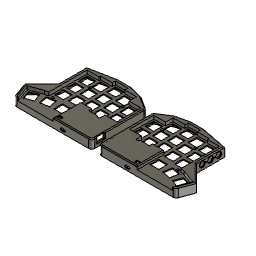
top_23333_3 (Autodesk Fusion 360 design; units mm, degrees)
Autodesk Fusion 360 part; units mm, degrees
sketch "case_plate_23333_3" plane through (0, 0, 0) normal (0, 0, 1) x (1, 0, 0)
  line L0 (133.9348, -86.7293) -> (107.5, -60.3353)
  line L1 (28.1017, -13.5688) -> (8.5, -25.9488)
  line L2 (126.2948, -107.72) -> (133.9348, -86.7293)
  line L3 (8.5, -107.72) -> (126.2948, -107.72)
  line L4 (8.5, -25.9488) -> (8.5, -107.72)
  line L5 (107.5, -60.3353) -> (107.5, -16.174)
  line L6 (67.6888, -8.518) -> (67.5953, -8.5)
  line L7 (67.5953, -8.5) -> (48.3769, -8.5)
  line L8 (107.5, -16.174) -> (67.6888, -8.518)
  line L9 (48.3769, -8.5) -> (28.1017, -13.5688)
  line L10 (128.3954, -110.72) -> (137.4081, -85.9579)
  line L11 (5.5, -110.72) -> (128.3954, -110.72)
  line L12 (110.5, -13.6959) -> (67.8811, -5.5)
  line L13 (5.5, -24.2953) -> (5.5, -110.72)
  line L14 (110.5, -59.0913) -> (110.5, -13.6959)
  line L15 (26.9069, -10.7752) -> (5.5, -24.2953)
  line L16 (48.0076, -5.5) -> (26.9069, -10.7752)
  line L17 (137.4081, -85.9579) -> (110.5, -59.0913)
  line L18 (67.8811, -5.5) -> (48.0076, -5.5)
  line L19 (135.3241, -86.4207) -> (108.7, -59.8377)
  line L20 (7.3, -25.2874) -> (7.3, -108.92)
  line L21 (27.6238, -12.4513) -> (7.3, -25.2874)
  line L22 (7.3, -108.92) -> (127.135, -108.92)
  line L23 (127.135, -108.92) -> (135.3241, -86.4207)
  line L24 (67.7096, -7.3) -> (48.2292, -7.3)
  line L25 (48.2292, -7.3) -> (27.6238, -12.4513)
  line L26 (108.7, -59.8377) -> (108.7, -15.1828)
  line L27 (108.7, -15.1828) -> (67.7096, -7.3)
  line L28 (109.3, -59.5889) -> (109.3, -14.6872)
  line L29 (68.0288, -6.7504) -> (67.7668, -6.7)
  line L30 (67.7668, -6.7) -> (48.1553, -6.7)
  line L31 (27.3848, -11.8926) -> (6.7, -24.9567)
  line L32 (136.0188, -86.2664) -> (109.3, -59.5889)
  line L33 (109.3, -14.6872) -> (68.0288, -6.7504)
  line L34 (127.5552, -109.52) -> (136.0188, -86.2664)
  line L35 (6.7, -24.9567) -> (6.7, -109.52)
  line L36 (48.1553, -6.7) -> (27.3848, -11.8926)
  line L37 (6.7, -109.52) -> (127.5552, -109.52)
  circle A0 centre (32, -34.5) radius 2.2
  circle A1 centre (84, -34.5) radius 2.2
  circle A2 centre (100.1356, -78.3241) radius 2.2
  line L38 (10.5, -104.61) -> (43.5, -104.61)
  line L39 (10.5, -86.61) -> (10.5, -104.61)
  line L40 (43.5, -104.61) -> (43.5, -86.61)
  line L41 (43.5, -86.61) -> (10.5, -86.61)
  line L42 (47.025, -101.99) -> (47.025, -107.84)
  line L43 (55.825, -107.84) -> (55.825, -101.99)
  line L44 (55.825, -101.99) -> (47.025, -101.99)
  line L45 (57.825, -106.475) -> (66.825, -106.475)
  line L46 (66.825, -102.975) -> (57.825, -102.975)
  line L47 (66.825, -106.475) -> (66.825, -102.975)
  line L48 (57.825, -102.975) -> (57.825, -106.475)
  line L49 (122.6064, -77.1718) -> (114.8282, -69.3936)
  line L50 (114.8282, -69.3936) -> (108.3936, -75.8282)
  line L51 (118.9049, -80.8732) -> (122.6064, -77.1718)
  line L52 (43.2, -83.45) -> (43.2, -74.55)
  line L53 (43.2, -74.55) -> (34.7125, -74.55)
  line L54 (34.6, -74.6909) -> (34.6, -83.45)
  line L55 (34.6, -83.45) -> (43.2, -83.45)
  line L56 (27, -63) -> (27, -49)
  line L57 (13, -63) -> (27, -63)
  line L58 (27, -49) -> (13, -49)
  line L59 (13, -49) -> (13, -63)
  line L60 (27, -30) -> (13, -30)
  line L61 (13, -30) -> (13, -44)
  line L62 (13, -44) -> (27, -44)
  line L63 (27, -44) -> (27, -30)
  line L64 (32, -70) -> (46, -70)
  line L65 (46, -70) -> (46, -56)
  line L66 (32, -56) -> (32, -70)
  line L67 (46, -56) -> (32, -56)
  line L68 (32, -51) -> (46, -51)
  line L69 (46, -37) -> (32, -37)
  line L70 (32, -37) -> (32, -51)
  line L71 (46, -51) -> (46, -37)
  line L72 (46, -18) -> (32, -18)
  line L73 (32, -18) -> (32, -32)
  line L74 (32, -32) -> (46, -32)
  line L75 (46, -32) -> (46, -18)
  line L76 (51, -51) -> (51, -65)
  line L77 (65, -65) -> (65, -51)
  line L78 (65, -51) -> (51, -51)
  line L79 (51, -65) -> (65, -65)
  line L80 (51, -32) -> (51, -46)
  line L81 (65, -46) -> (65, -32)
  line L82 (51, -46) -> (65, -46)
  line L83 (65, -32) -> (51, -32)
  line L84 (65, -27) -> (65, -13)
  line L85 (51, -13) -> (51, -27)
  line L86 (65, -13) -> (51, -13)
  line L87 (51, -27) -> (65, -27)
  line L88 (70, -70) -> (84, -70)
  line L89 (84, -70) -> (84, -56)
  line L90 (84, -56) -> (70, -56)
  line L91 (70, -56) -> (70, -70)
  line L92 (70, -37) -> (70, -51)
  line L93 (84, -51) -> (84, -37)
  line L94 (70, -51) -> (84, -51)
  line L95 (84, -37) -> (70, -37)
  line L96 (70, -32) -> (84, -32)
  line L97 (84, -18) -> (70, -18)
  line L98 (70, -18) -> (70, -32)
  line L99 (84, -32) -> (84, -18)
  line L100 (89, -58.5) -> (89, -72.5)
  line L101 (103, -72.5) -> (103, -58.5)
  line L102 (103, -58.5) -> (89, -58.5)
  line L103 (89, -72.5) -> (103, -72.5)
  line L104 (89, -39.5) -> (89, -53.5)
  line L105 (89, -53.5) -> (103, -53.5)
  line L106 (103, -39.5) -> (89, -39.5)
  line L107 (103, -53.5) -> (103, -39.5)
  line L108 (89, -34.5) -> (103, -34.5)
  line L109 (89, -20.5) -> (89, -34.5)
  line L110 (103, -34.5) -> (103, -20.5)
  line L111 (103, -20.5) -> (89, -20.5)
  line L112 (70, -78.8) -> (70, -92.8)
  line L113 (84, -92.8) -> (84, -78.8)
  line L114 (70, -92.8) -> (84, -92.8)
  line L115 (84, -78.8) -> (70, -78.8)
  line L116 (92.8078, -79.5706) -> (90.3767, -93.3579)
  line L117 (90.3767, -93.3579) -> (104.164, -95.789)
  line L118 (106.5951, -82.0017) -> (92.8078, -79.5706)
  line L119 (104.164, -95.789) -> (106.5951, -82.0017)
  line L120 (110.347, -97.4457) -> (123.5027, -102.234)
  line L121 (115.1353, -84.29) -> (110.347, -97.4457)
  line L122 (128.291, -89.0783) -> (115.1353, -84.29)
  line L123 (123.5027, -102.234) -> (128.291, -89.0783)
  line L124 (8.5, -65.75) -> (29.25, -65.75)
  line L125 (10.25, -65.75) -> (10.25, -27.25)
  line L126 (29.25, -27.25) -> (10.25, -27.25)
  line L127 (48.75, -72.75) -> (48.75, -67.75)
  line L128 (29.25, -65.75) -> (29.25, -72.75)
  line L129 (48.25, -15.25) -> (29.25, -15.25)
  line L130 (29.25, -15.25) -> (29.25, -27.25)
  line L131 (48.75, -67.75) -> (67.25, -67.75)
  line L132 (67.75, -15.25) -> (67.75, -10.25)
  line L133 (67.75, -10.25) -> (48.25, -10.25)
  line L134 (48.25, -10.25) -> (48.25, -15.25)
  line L135 (67.25, -110.72) -> (67.25, -67.75)
  line L136 (86.75, -17.75) -> (86.75, -15.25)
  line L137 (86.75, -15.25) -> (67.75, -15.25)
  line L138 (105.75, -60.3353) -> (105.75, -17.75)
  line L139 (105.75, -17.75) -> (86.75, -17.75)
  line L140 (67.25, -95.55) -> (86.9722, -95.55)
  line L141 (86.9722, -95.55) -> (106.6135, -99.0133)
  line L142 (105.75, -79.0602) -> (111.608, -80.0931)
  line L143 (106.6135, -99.0133) -> (125.1463, -105.7587)
  line L144 (123.3406, -110.72) -> (131.8157, -87.4347)
  line L145 (111.7483, -80.1307) -> (133.4602, -88.0332)
  line L146 (107.5, -60.3353) -> (105.75, -60.3353)
  line L147 (105.75, -79.0602) -> (105.75, -60.3353)
  arc A3 (32, -74.7) -> (34.1857, -72.75) centre (32, -72.5) ccw
  line L148 (34.1857, -72.75) -> (48.75, -72.75)
  line L149 (32, -74.7) -> (29.25, -74.7)
  line L150 (29.25, -74.7) -> (29.25, -72.75)
  line L151 (8.5, -66.95) -> (28.05, -66.95)
  line L152 (28.05, -66.95) -> (28.05, -72.75)
  line L153 (28.05, -75.9) -> (28.05, -72.75)
  line L154 (32, -75.9) -> (28.05, -75.9)
  arc A4 (32, -75.9) -> (35.0753, -73.95) centre (32, -72.5) ccw
  line L155 (35.0753, -73.95) -> (49.95, -73.95)
  line L156 (49.95, -73.95) -> (49.95, -68.95)
  line L157 (49.95, -68.95) -> (66.05, -68.95)
  line L158 (66.05, -110.72) -> (66.05, -68.95)
  line L159 (111.608, -80.0931) -> (111.7483, -80.1307)
  line L160 (107.5, -77.5918) -> (107.5, -60.3353)
  line L161 (107.5, -77.5918) -> (111.9871, -78.383)
  line L162 (111.9871, -78.383) -> (112.275, -78.4601)
  line L163 (112.275, -78.4601) -> (134.0587, -86.3888)
  line L164 (108.3936, -75.8282) -> (110.7259, -78.1606)
extrude "Extrude1" add sketch "case_plate_23333_3" along normal blind 1.6 contours L124 L125 L126 L127 L128 L129 L130 L131 L132 L133 L134 L135 L136 L137 L138 L139 L140 L141 L142 L143 L144 L145 L147 A3 L148 L149 L150 L159 | L3 L22 L135 L144 | L3 L135 L140 L141 L143 L144 | L22 L37 L135 L144 | L11 L37 L135 L144 | A0 | A1 | A2 makes body 1
extrude "Extrude2" add sketch "case_plate_23333_3" along normal blind 7 contours L0 L2 L142 L145 L146 L147 L159 L160 L161 L162 L163 | L0 L1 L2 L3 L4 L5 L6 L7 L8 L9 L19 L20 L21 L22 L23 L24 L25 L26 L27 L144 L158 | L2 L3 L144 L145 | L1 L4 L5 L6 L7 L8 L9 L124 L125 L126 L129 L130 L132 L133 L134 L136 L137 L138 L139 L146 | L3 L22 L135 L158 | L3 L4 L45 L46 L47 L124 L127 L128 L131 L135 A3 L148 L149 L150 L151 L152 L153 L154 A4 L155 L156 L157 L158 | L19 L20 L21 L22 L23 L24 L25 L26 L27 L28 L29 L30 L31 L32 L33 L34 L35 L36 L37 L144 L158 | L22 L37 L135 L158 | L10 L11 L12 L13 L14 L15 L16 L17 L18 L28 L29 L30 L31 L32 L33 L34 L35 L36 L37 L144 L158 | L45 L46 L47 L158 | L11 L37 L135 L158 bodies 1
extrude "Extrude3" add sketch "case_plate_23333_3" along normal blind 1.6 from surface at 5.4 contours L0 L49 L50 L51 L160 L161 L163 L164 | L49 L50 L51 L161 L162 L163 L164 | L3 L4 L42 L43 L44 L45 L46 L48 L52 L53 L54 L55 L151 L152 L153 L154 A4 L155 L156 L157 L158 | L3 L42 L43 L44 | L45 L46 L48 L158 | L52 L53 L54 L55 A4 | L38 L39 L40 L41 bodies 1
extrude "Extrude4" add sketch "case_plate_23333_3" against normal blind 6.8 contours L0 L1 L2 L3 L4 L5 L6 L7 L8 L9 L19 L20 L21 L22 L23 L24 L25 L26 L27 L144 L158 | L3 L22 L135 L144 | L3 L22 L135 L158 | L22 L37 L135 L144 | L19 L20 L21 L22 L23 L24 L25 L26 L27 L28 L29 L30 L31 L32 L33 L34 L35 L36 L37 L144 L158 | L22 L37 L135 L158 bodies 1
extrude "Extrude5" add sketch "case_plate_23333_3" against normal blind 7.6 contours L11 L37 L135 L144 | L10 L11 L12 L13 L14 L15 L16 L17 L18 L28 L29 L30 L31 L32 L33 L34 L35 L36 L37 L144 L158 | L11 L37 L135 L158 bodies 1
move_body "Move2" bodies 1 to x (1, 0, 0) y (0, 1, 0) z (0, 0, 1) at (0, 0, -1.6)
hole "Hole1" at (84, -34.5, 0) at (100.1356, -78.3241, 0) at (32, -72.5, 0) at (32, -34.5, 0) direction (0, 0, -1) diameter 2.4 depth 25 tip angle 118 countersink diameter 4.4 countersink angle 90 bodies 1
sketch "usb" plane through (5.5, 0, 0) normal (-1, 0, 0) x (0, -1, 0)
  line L0 (110.72, -9.2) -> (110.72, 5.4)
  line L1 (110.72, 5.4) -> (24.2953, 5.4)
  line L2 (24.2953, 5.4) -> (24.2953, -9.2)
  line L3 (24.2953, -9.2) -> (110.72, -9.2)
  line L4 (86.61, 0) -> (104.61, 0) construction
  line L5 (87.9038, 4.2) -> (106.2348, 4.2)
  line L6 (87.9913, -3.8) -> (106.3223, -3.8)
  line L7 (89.61, 4.2) -> (89.61, -3.8)
  line L8 (101.61, 4.2) -> (101.61, -3.8)
  dimension "d17" = 1.2
  dimension "d18" = 8
  dimension "d19" = 3
  dimension "d20" = 12
  constraint parallel L1 L5
  constraint parallel L4 L6
  constraint coincident L5 L7.start
  constraint coincident L6 L7.end
  constraint perpendicular L6 L7
  constraint coincident L5 L8.start
  constraint coincident L6 L8.end
  constraint perpendicular L6 L8
  measures "d17" distance of L1 L5
  measures "d18" distance of L5 L6
  measures "d19" distance of L4.start L7
  measures "d20" distance of L7 L8
extrude "Extrude6" cut sketch "usb" against normal up to surface (3 mm away) contours L5 L6 L7 L8 bodies 1
chamfer "Chamfer1" distance 1 angle 45 4 edges at (5.5, -95.61, 4.2) (5.5, -89.61, 0.2) (5.5, -95.61, -3.8) (5.5, -101.61, 0.2) on bodies 1
sketch "pwr" plane through (0, -110.72, 0) normal (0, -1, 0) x (1, 0, 0)
  line L0 (128.3954, -9.2) -> (128.3954, 5.4)
  line L1 (128.3954, 5.4) -> (123.3406, 5.4)
  line L2 (123.3406, 5.4) -> (123.3406, 0)
  line L3 (123.3406, 0) -> (67.25, 0)
  line L4 (67.25, 0) -> (67.25, 5.4)
  line L5 (67.25, 5.4) -> (5.5, 5.4)
  line L6 (5.5, 5.4) -> (5.5, -9.2)
  line L7 (5.5, -9.2) -> (128.3954, -9.2)
  line L8 (55.825, 0) -> (47.025, 0) construction
  line L9 (42.4021, -5) -> (67.724, -5) construction
  line L10 (40.3061, -4.25) -> (71.2929, -4.25) construction
  line L11 (49.425, -4.25) -> (49.425, 0) construction
  line L12 (53.425, 0) -> (53.425, -4.25) construction
  line L13 (49.425, -5.75) -> (53.425, -5.75)
  arc A0 (53.425, -5.75) -> (53.425, -2.75) centre (53.425, -4.25) ccw
  line L14 (53.425, -2.75) -> (49.425, -2.75)
  arc A1 (49.425, -2.75) -> (49.425, -5.75) centre (49.425, -4.25) ccw
  line L15 (49.425, -4.25) -> (53.425, -4.25) construction
  dimension "d24" = 10.4
  dimension "d25" = 0.75
  dimension "d26" = 2.4
  dimension "d27" = 4
  dimension "d28" = 3
  constraint horizontal L9
  constraint parallel L9 L10
  constraint coincident L10 L11.start
  constraint coincident L8 L11.end
  constraint perpendicular L8 L11
  constraint coincident L8 L12.start
  constraint coincident L10 L12.end
  constraint perpendicular L10 L12
  constraint tangent L13 A0
  constraint tangent A0 L14
  constraint parallel L13 L14
  constraint tangent L14 A1
  constraint tangent L13 A1
  constraint coincident L12.end A0.centre
  constraint perpendicular L12 L15
  constraint coincident L11.start A1.centre
  measures "d24" distance of L5 L9
  measures "d25" distance of L9 L10
  measures "d26" distance of L8.end L11
  measures "d27" distance of L11 L12
  measures "d28" diameter of A0
extrude "Extrude7" cut sketch "pwr" against normal up to surface (3 mm away) contours L13 A0 L14 A1 bodies 1
sketch "Sketch4" plane through (0, 0, -5.75) normal (0, 0, 1) x (-1, 0, 0)
  line L0 (-49.425, 110.72) -> (-53.425, 110.72)
  line L1 (-53.425, 110.72) -> (-53.425, 107.72)
  line L2 (-53.425, 107.72) -> (-49.425, 107.72)
  line L3 (-49.425, 107.72) -> (-49.425, 110.72)
  line L4 (-49.425, 109.22) -> (-53.425, 109.22)
  constraint midpoint L3 L4.start
  constraint midpoint L1 L4.end
extrude "Extrude8" cut sketch "Sketch4" against normal up to surface (2.65 mm away) contours L1 L2 L3 L4 bodies 1
chamfer "Chamfer2" distance 0.5 angle 45 4 edges at (51.425, -110.72, -2.75) (54.925, -110.72, -4.25) (51.425, -110.72, -5.75) (47.925, -110.72, -4.25) on bodies 1
sketch "Sketch5" plane through (0, 0, 5.4) normal (0, 0, 1) x (-1, 0, 0)
  line L0 (-105.75, 79.0602) -> (-111.608, 80.0931)
  line L1 (-111.608, 80.0931) -> (-111.7483, 80.1307)
  line L2 (-111.7483, 80.1307) -> (-131.8157, 87.4347)
  line L3 (-131.8157, 87.4347) -> (-123.3406, 110.72)
  line L4 (-123.3406, 110.72) -> (-128.3954, 110.72)
  line L5 (-128.3954, 110.72) -> (-137.4081, 85.9579)
  line L6 (-137.4081, 85.9579) -> (-110.5, 59.0913)
  line L7 (-110.5, 59.0913) -> (-110.5, 13.6959)
  line L8 (-110.5, 13.6959) -> (-67.8811, 5.5)
  line L9 (-67.8811, 5.5) -> (-48.0076, 5.5)
  line L10 (-48.0076, 5.5) -> (-26.9069, 10.7752)
  line L11 (-26.9069, 10.7752) -> (-5.5, 24.2953)
  line L12 (-5.5, 24.2953) -> (-5.5, 110.72)
  line L13 (-5.5, 110.72) -> (-67.25, 110.72)
  line L14 (-67.25, 110.72) -> (-67.25, 67.75)
  line L15 (-67.25, 67.75) -> (-48.75, 67.75)
  line L16 (-48.75, 67.75) -> (-48.75, 72.75)
  line L17 (-48.75, 72.75) -> (-34.1857, 72.75)
  arc A0 (-32, 74.7) -> (-34.1857, 72.75) centre (-32, 72.5) ccw
  line L18 (-32, 74.7) -> (-29.25, 74.7)
  line L19 (-29.25, 74.7) -> (-29.25, 65.75)
  line L20 (-29.25, 65.75) -> (-10.25, 65.75)
  line L21 (-10.25, 65.75) -> (-10.25, 27.25)
  line L22 (-10.25, 27.25) -> (-29.25, 27.25)
  line L23 (-29.25, 27.25) -> (-29.25, 15.25)
  line L24 (-29.25, 15.25) -> (-48.25, 15.25)
  line L25 (-48.25, 15.25) -> (-48.25, 10.25)
  line L26 (-48.25, 10.25) -> (-67.75, 10.25)
  line L27 (-67.75, 10.25) -> (-67.75, 15.25)
  line L28 (-67.75, 15.25) -> (-86.75, 15.25)
  line L29 (-86.75, 15.25) -> (-86.75, 17.75)
  line L30 (-86.75, 17.75) -> (-105.75, 17.75)
  line L31 (-105.75, 17.75) -> (-105.75, 79.0602)
  line L32 (-66.825, 102.975) -> (-57.825, 102.975)
  line L33 (-57.825, 102.975) -> (-57.825, 106.475)
  line L34 (-57.825, 106.475) -> (-66.825, 106.475)
  line L35 (-66.825, 106.475) -> (-66.825, 102.975)
  line L36 (-59.325, 102.975) -> (-59.325, 106.475)
  line L37 (-65.325, 102.975) -> (-65.325, 106.475)
  dimension "d34" = 1.5
  dimension "d35" = 1.5
  constraint coincident L32 L36.start
  constraint coincident L34 L36.end
  constraint perpendicular L34 L36
  constraint coincident L32 L37.start
  constraint coincident L34 L37.end
  constraint perpendicular L34 L37
  measures "d34" distance of L33 L36
  measures "d35" distance of L35 L37
extrude "Extrude9" cut sketch "Sketch5" against normal up to surface (1.6 mm away) contours L32 L34 L36 L37 bodies 1
chamfer "Chamfer3" distance 0.4 angle 45 4 edges at (62.325, -102.975, 5.4) (59.325, -104.725, 5.4) (62.325, -106.475, 5.4) (65.325, -104.725, 5.4) on bodies 1
sketch "Sketch6" plane through (110.5, 0, 0) normal (1, 0, 0) x (0, 1, 0)
  line L0 (-13.6959, -9.2) -> (-13.6959, 5.4)
  line L1 (-13.6959, 5.4) -> (-59.0913, 5.4)
  line L2 (-59.0913, 5.4) -> (-59.0913, -9.2)
  line L3 (-59.0913, -9.2) -> (-13.6959, -9.2)
  line L4 (-59.0913, -9.2) -> (-13.6959, -9.2)
  line L5 (-13.6959, 5.4) -> (-59.0913, 5.4)
  line L6 (-59.0913, 5.4) -> (-59.0913, -9.2)
  line L7 (-13.6959, -9.2) -> (-13.6959, 5.4)
  line L8 (-51.6694, 2.486) -> (-53.9835, -1.4778)
  line L9 (-51.7078, -5.4639) -> (-47.1179, -5.486)
  line L10 (-47.1179, -5.486) -> (-44.8038, -1.5222)
  line L11 (-44.8038, -1.5222) -> (-47.0795, 2.4639)
  line L12 (-53.9835, -1.4778) -> (-51.7078, -5.4639)
  line L13 (-47.0795, 2.4639) -> (-51.6694, 2.486)
  line L14 (-31.8038, -1.5222) -> (-34.0795, 2.4639)
  line L15 (-40.9835, -1.4778) -> (-38.7078, -5.4639)
  line L16 (-34.0795, 2.4639) -> (-38.6694, 2.486)
  line L17 (-38.7078, -5.4639) -> (-34.1179, -5.486)
  line L18 (-34.1179, -5.486) -> (-31.8038, -1.5222)
  line L19 (-38.6694, 2.486) -> (-40.9835, -1.4778)
  line L20 (-21.0795, 2.4639) -> (-25.6694, 2.486)
  line L21 (-25.6694, 2.486) -> (-27.9835, -1.4778)
  line L22 (-21.1179, -5.486) -> (-18.8038, -1.5222)
  line L23 (-18.8038, -1.5222) -> (-21.0795, 2.4639)
  line L24 (-25.7078, -5.4639) -> (-21.1179, -5.486)
  line L25 (-27.9835, -1.4778) -> (-25.7078, -5.4639)
  arc A0 (-49.3936, -0.75) -> (-49.3936, -2.25) centre (-49.3936, -1.5) ccw
  arc A1 (-23.3936, -2.25) -> (-23.3936, -0.75) centre (-23.3936, -1.5) ccw
  line L26 (-49.3936, -2.25) -> (-23.3936, -2.25)
  line L27 (-23.3936, -0.75) -> (-49.3936, -0.75)
  line L28 (-59.0913, -1.5) -> (-13.6959, -1.5) construction
  line L29 (-49.3936, -1.5) -> (-23.3936, -1.5) construction
  point P0 (-36.3936, -1.5)
  point P1 (-49.3936, -1.5)
  point P2 (-36.3936, -1.5)
  point P3 (-23.3936, -1.5)
extrude "Extrude10" cut sketch "Sketch6" against normal blind 2 contours L8 L9 L10 L11 L12 L13 A0 L26 L27 | L10 L11 L15 L19 L26 L27 | L10 L11 A0 L26 L27 | L14 L15 L18 L19 L26 L27 | L14 L16 L19 L27 | L14 L18 L21 L25 L26 L27 | L15 L17 L18 L26 | L21 L25 A1 L26 L27 | L20 L21 L22 L23 L24 L25 A1 L26 L27 bodies 1
sketch "Sketch7" plane through (25.619, 25.6586, 0) normal (0.70656, 0.707653, 0) x (-0.707653, 0.70656, 0)
  line L0 (-119.9472, -9.2) -> (-119.9472, 5.4)
  line L1 (-119.9472, 5.4) -> (-157.9716, 5.4)
  line L2 (-157.9716, 5.4) -> (-157.9716, -9.2)
  line L3 (-157.9716, -9.2) -> (-119.9472, -9.2)
  line L4 (-139.2893, -5.5) -> (-139.2893, -4.5)
  line L5 (-139.2893, -4.5) -> (-132.2893, -4.5)
  line L6 (-132.2893, -4.5) -> (-132.2893, -5.5)
  line L7 (-132.2893, -5.5) -> (-139.2893, -5.5)
  line L8 (-157.9716, -9.2) -> (-119.9472, -9.2)
  line L9 (-157.9716, 5.4) -> (-157.9716, -9.2)
  line L10 (-119.9472, 5.4) -> (-157.9716, 5.4)
  line L11 (-119.9472, -9.2) -> (-119.9472, 5.4)
  line L12 (-148.2729, -5.4713) -> (-143.683, -5.4786)
  line L13 (-143.6704, 2.4713) -> (-148.2603, 2.4786)
  line L14 (-141.3817, -1.5073) -> (-143.6704, 2.4713)
  line L15 (-143.683, -5.4786) -> (-141.3817, -1.5073)
  line L16 (-148.2603, 2.4786) -> (-150.5616, -1.4927)
  line L17 (-150.5616, -1.4927) -> (-148.2729, -5.4713)
  line L18 (-125.646, -5.4713) -> (-123.3573, -1.4927)
  line L19 (-130.2485, 2.4713) -> (-132.5372, -1.5073)
  line L20 (-132.5372, -1.5073) -> (-130.2359, -5.4786)
  line L21 (-125.6586, 2.4786) -> (-130.2485, 2.4713)
  line L22 (-130.2359, -5.4786) -> (-125.646, -5.4713)
  line L23 (-123.3573, -1.4927) -> (-125.6586, 2.4786)
  line L24 (-145.9716, -2.25) -> (-127.9472, -2.25)
  line L25 (-127.9472, -0.75) -> (-145.9716, -0.75)
  arc A0 (-145.9716, -0.75) -> (-145.9716, -2.25) centre (-145.9716, -1.5) ccw
  arc A1 (-127.9472, -2.25) -> (-127.9472, -0.75) centre (-127.9472, -1.5) ccw
  line L26 (-157.9716, -1.5) -> (-119.9472, -1.5) construction
  line L27 (-145.9716, -1.5) -> (-127.9472, -1.5) construction
  point P0 (-145.9716, -1.5)
  point P1 (-127.9472, -1.5)
extrude "Extrude11" cut sketch "Sketch7" against normal blind 2 contours L12 L13 L14 L15 L16 L17 L24 L25 A0 | L14 L15 L24 L25 A0 | L14 L15 L19 L20 L24 L25 | L18 L19 L20 L21 L22 L23 L24 L25 A1 | L19 L20 L24 L25 A1 bodies 1
extrude "Extrude12" cut sketch "Sketch7" against normal up to surface (3 mm away) contours L4 L5 L6 L7 bodies 1
chamfer "Chamfer4" distance 0.4 angle 45 30 edges at (131.3501, -79.9092, 0.493) (128.9118, -77.4747, 2.475) (131.3545, -79.9137, -3.482) (128.9207, -77.4836, -5.475) (126.6347, -75.2011, -3.8643) (126.6321, -75.1985, 0.8607) (118.4454, -67.0244, 0.8607) (116.1657, -64.7483, 2.475) (113.7274, -62.3138, 0.493) (113.7229, -62.3093, -3.482) (116.1568, -64.7393, -5.475) (118.4428, -67.0218, -3.8643) (110.5, -49.3744, 2.475) (110.5, -52.8265, 0.5041) (110.5, -52.8456, -3.4709) (110.5, -49.4128, -5.475) (110.5, -46.1733, -3.868) (110.5, -46.1621, 0.8569) (110.5, -39.614, 0.868) (110.5, -39.6252, -3.8569) (110.5, -36.4128, -5.475) (110.5, -33.1733, -3.868) (110.5, -33.1621, 0.8569) (110.5, -36.3744, 2.475) (110.5, -26.614, 0.868) (110.5, -26.6252, -3.8569) (110.5, -23.4128, -5.475) (110.5, -23.3744, 2.475) (110.5, -19.9416, 0.4709) (110.5, -19.9608, -3.5041) on bodies 1
fillet "Fillet1" radius 2 6 edges at (67.5953, -8.5, -5) (48.3769, -8.5, -5) (28.1017, -13.5688, -5) (8.5, -25.9488, -5) (8.5, -107.72, -2.3) (126.2948, -107.72, -5) on bodies 1
fillet "Fillet2" radius 5 12 edges at (67.7668, -6.7, -8.8) (48.1553, -6.7, -8.8) (27.3848, -11.8926, -8.8) (6.7, -24.9567, -8.8) (6.7, -109.52, -8.8) (127.5552, -109.52, -8.8) (128.3954, -110.72, -1.9) (5.5, -110.72, -1.9) (5.5, -24.2953, -1.9) (26.9069, -10.7752, -1.9) (48.0076, -5.5, -1.9) (67.8811, -5.5, -1.9) on bodies 1
chamfer "Chamfer5" distance 1.5 angle 45 18 edges at (38.875, -110.72, 5.4) (6.9645, -109.2555, 5.4) (5.5, -66.3856, 5.4) (6.1211, -24.6376, 5.4) (17.0292, -17.0137, 5.4) (26.9321, -10.834, 5.4) (37.548, -8.1149, 5.4) (48.0122, -5.5375, 5.4) (58.0139, -5.5, 5.4) (67.879, -5.5225, 5.4) (89.4245, -9.643, 5.4) (110.5, -36.3936, 5.4) (123.954, -72.5246, 5.4) (133.5005, -96.694, 5.4) (127.7623, -109.8157, 5.4) (124.1175, -110.72, 5.4) (127.5781, -99.0773, 5.4) (67.25, -89.235, 5.4) on bodies 1
mirror "Mirror1" about plane through (0, 0, 0) normal (1, 0, 0) of bodies 1 makes body 2
